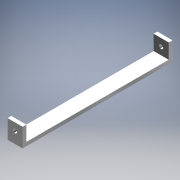
# Autodesk Inventor part: Back Support Piece
Saved by Autodesk Inventor 2019.4 (Build 234330000, 330)
## iProperties
Created: 2020-01-18
Part Number: Back Support Piece
Material: Aluminum 6061
Document SubType Name: Sheet Metal
Designer: Mark
Mass: 64.1585 g
Surface Area: 122.778 cm^2
Volume: 23.7624 cm^3
Density: 2.7 g/cm^3
Sheet Metal Rule: Default_mm
Appearance: Aluminum - Flat
Author: Mark
Autodesk Inventor part; units mm, degrees
ref_plane "YZ Plane" through (0, 0, 0) normal (1, 0, 0) x (0, 1, 0)
ref_plane "XZ Plane" through (0, 0, 0) normal (0, 1, 0) x (-1, 0, 0)
ref_plane "XY Plane" through (0, 0, 0) normal (0, 0, 1) x (1, 0, 0)
sketch "Sketch1" plane through (0, 0, 0) normal (1, 0, 0) x (0, 1, 0)
  line L0 (69.8276, 510.5354) -> (64.8276, 510.5354)
  line L1 (64.8276, 510.5354) -> (64.8276, 310.5354)
  line L2 (64.8276, 310.5354) -> (69.8276, 310.5354)
  line L3 (69.8276, 310.5354) -> (69.8276, 510.5354)
  point P0 (0, 0)
  dimension "d0" = 5
  dimension "d1" = 200
  constraints: 8 end point, 2 parallel, 1 horizontal, 1 perpendicular
  measures "d0" distance of L2.end L1.end
  measures "d1" distance of L1.end L0.end
extrude "Extrusion1" add sketch "Sketch1" along normal blind 20
sketch "Sketch2" plane through (0, 69.8276, 510.5354) normal (0, 1, 0) x (1, 0, 0)
  line L0 (20, 0) -> (20, 200) projected
  line L1 (0, 0) -> (0, 200) projected
  line L2 (20, 200) -> (0, 200)
  line L3 (0, 200) -> (0, 195)
  line L4 (0, 195) -> (20, 195)
  line L5 (20, 195) -> (20, 200)
  line L6 (0, 0) -> (20, 0) projected
  line L7 (0, 0) -> (20, 0)
  line L8 (20, 0) -> (20, 5)
  line L9 (20, 5) -> (0, 5)
  line L10 (0, 5) -> (0, 0)
  point P0 (0, 510.5354)
  dimension "d4" = 5
  dimension "d5" = 5
  constraints: 16 end point, 4 parallel, 2 horizontal, 2 perpendicular, 2 point on line
  measures "d4" distance of L3.end L2.end
  measures "d5" distance of L8.end L7.end
extrude "Extrusion2" add sketch "Sketch2" along normal blind 20 contours L6 L1 L9 L0 | L4 L1 L2 L0
sketch "Sketch3" plane through (0, 64.8276, 510.5354) normal (0, 0, 1) x (1, 0, 0)
  circle A0 centre (10, 15) radius 2.75
  line L0 (20, 0) -> (20, 25) projected
  line L1 (0, 25) -> (20, 25) projected
  point P0 (0, -64.8276)
  dimension "d8" = 5.5
  dimension "d9" = 10
  dimension "d10" = 10
  constraints: 1 centre point
  measures "d8" diameter of A0
  measures "d9" distance from line of L0 A0.centre
  measures "d10" distance from line of L1 A0.centre
extrude "Extrusion3" cut sketch "Sketch3" against normal blind 200
equation "\"BendRadius\" = Thickness"
equation "\"BendReliefWidth\" = Thickness"
equation "\"BendReliefDepth\" = 0.5 * Thickness"
equation "\"CornerReliefSize\" = 4 * Thickness"
equation "\"MinimumRemnant\" = 2 * Thickness"
equation "\"TransitionRadius\" = BendRadius"
equation "\"JacobiRadiusSize\" = BendRadius"
equation "\"GapSize\" = Thickness"
equation "\"Thickness\" = 0.5"
body "Solid1"
